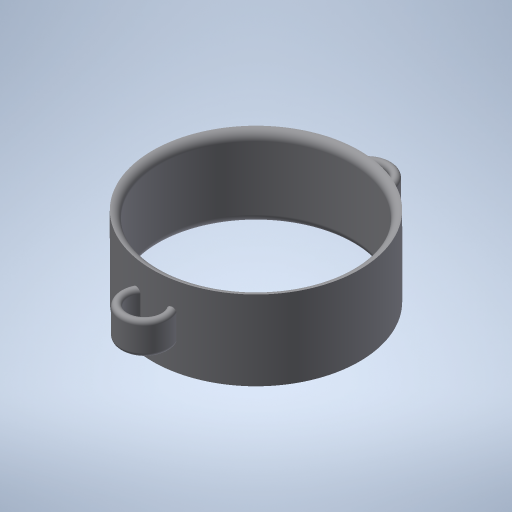
# Autodesk Inventor part: anillos
Saved by Autodesk Inventor 2023 (Build 270158000, 158)
## iProperties
Created: 2022-10-17
Part Number: anillos
Material: Generic
Document SubType Name: Modeling
Designer: Xiaba
Density: 1 g/cm^3
Appearance: Default
Author: Xiaba
Autodesk Inventor part; units mm, degrees
ref_plane "YZ Plane" through (0, 0, 0) normal (1, 0, 0) x (0, 1, 0)
ref_plane "XZ Plane" through (0, 0, 0) normal (0, 1, 0) x (-1, 0, 0)
ref_plane "XY Plane" through (0, 0, 0) normal (0, 0, 1) x (1, 0, 0)
sketch "Sketch1" plane through (0, 0, 0) normal (0, 1, 0) x (-1, 0, 0)
  circle A0 centre (0, 0) radius 6
  circle A1 centre (0, 0) radius 6.5
  dimension "d0" = 12
  dimension "d1" = 13
  constraints: 2 centre point, 2 coincident
  measures "d0" diameter of A0
  measures "d1" diameter of A1
extrude "Extrusion1" add sketch "Sketch1" along normal blind 5
sketch "Sketch2" plane through (0, 5, 0) normal (0, 1, 0) x (1, 0, 0)
  circle A0 centre (0, -7) radius 1
  circle A1 centre (0, 0) radius 6 projected
  circle A2 centre (0, -7) radius 1.5
  circle A3 centre (0, 7) radius 1
  circle A4 centre (0, 7) radius 1.5
  dimension "d4" = 2
  dimension "d5" = 3
  dimension "d6" = 2
  dimension "d7" = 3
  constraints: 4 centre point, 2 coincident, 2 tangent
  measures "d4" diameter of A0
  measures "d5" diameter of A2
  measures "d6" diameter of A3
  measures "d7" diameter of A4
sketch "Sketch3" plane through (0, 5, 0) normal (0, 1, 0) x (1, 0, 0)
  circle A0 centre (0, 0) radius 6 projected
extrude "Extrusion2" add sketch "Sketch2" against normal blind 5 contours A1 A2 | A1 A2 | A4 A1 | A1 A4
extrude "Extrusion3" cut sketch "Sketch3" against normal through all
sketch "Sketch4" plane through (0, 5, 0) normal (0, 1, 0) x (1, 0, 0)
  arc A0 (-1.3553, -6.3571) -> (1.3553, -6.3571) centre (0, -7) ccw projected
  arc A1 (-0.8328, -6.4464) -> (0.8328, -6.4464) centre (0, -7) ccw projected
  arc A2 (1.3553, 6.3571) -> (-1.3553, 6.3571) centre (0, 7) ccw projected
  arc A3 (0.8328, 6.4464) -> (-0.8328, 6.4464) centre (0, 7) ccw projected
  circle A4 centre (0, 0) radius 6
  arc A5 (1.3553, -6.3571) -> (1.3553, 6.3571) centre (0, 0) ccw projected
  circle A6 centre (0, 0) radius 6.5
  point P0 (-1.3553, 6.3571)
  point P1 (-0.8328, 6.4464)
  point P2 (-1.3553, -6.3571)
  point P3 (0.8328, -6.4464)
  constraints: 2 coincident, 1 centre point, 3 other
extrude "Extrusion4" cut sketch "Sketch4" against normal blind 1.5 contours A6 A1 A0 | A2 A6 A3
sketch "Sketch5" plane through (0, 0, 0) normal (0, -1, 0) x (1, 0, 0)
  arc A0 (1.3553, 6.3571) -> (-1.3553, 6.3571) centre (0, 7) ccw projected
  arc A1 (-1.3553, -6.3571) -> (1.3553, -6.3571) centre (0, -7) ccw projected
  circle A2 centre (0, 0) radius 6.5
  arc A3 (0.8328, 6.4464) -> (-0.8328, 6.4464) centre (0, 7) ccw projected
  arc A4 (-0.8328, -6.4464) -> (0.8328, -6.4464) centre (0, -7) ccw projected
  point P0 (1.3553, -6.3571)
  point P1 (1.3553, 6.3571)
  constraints: 1 centre point, 1 coincident, 1 point on circle
extrude "Extrusion5" cut sketch "Sketch5" against normal blind 1.5 contours A2 A3 A0 | A2 A4 A1
fillet "Fillet1" radius 0.25 8 edges at (0, 3.5, 8.5) (0, 1.5, 8.5) (0, 3.5, 8) (0, 1.5, 8) (0, 3.5, -8.5) (0, 3.5, -8) (0, 1.5, -8) (0, 1.5, -8.5)
fillet "Fillet2" radius 0.5 2 edges at (-1.0312, 5, -5.9107) (-1.0312, 0, -5.9107)
body "Solid1"
